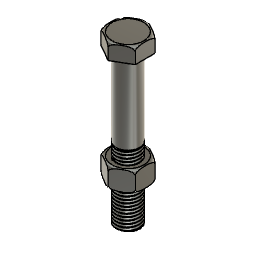
Part 5_ Modelling Features v2 (Autodesk Fusion 360 design; units mm, degrees)
Autodesk Fusion 360 part; units mm, degrees
sketch "Sketch1" plane through (0, 0, 0) normal (0, 0, 1) x (1, 0, 0)
  circle A0 centre (0, 0) radius 6
  line L0 (0, 10) -> (-8.6603, 5)
  line L1 (-8.6603, 5) -> (-8.6603, -5)
  line L2 (-8.6603, -5) -> (0, -10)
  line L3 (0, -10) -> (8.6603, -5)
  line L4 (8.6603, -5) -> (8.6603, 5)
  line L5 (8.6603, 5) -> (0, 10)
  dimension "d1" = 12
  dimension "d2" = 10
  constraint coincident A0.centre origin
  constraint vertical L4
  measures "d1" diameter of A0
  measures "d2" distance of L0.start A0.centre
extrude "Extrude1" add sketch "Sketch1" along normal blind 76 contours A0 makes body 1
extrude "Extrude2" add sketch "Sketch1" along normal blind 7.6 from surface at 76 contours A0 | L0 L1 L2 L3 L4 L5 bodies 1
sketch "Sketch4" plane through (0, 0, 83.6) normal (0, 0, 1) x (-1, 0, 0)
  line L0 (-8.6603, 5) -> (-8.6603, -5)
  line L1 (-8.6603, -5) -> (0, -10)
  line L2 (0, -10) -> (8.6603, -5)
  line L3 (8.6603, -5) -> (8.6603, 5)
  line L4 (8.6603, 5) -> (0, 10)
  line L5 (0, 10) -> (-8.6603, 5)
  circle A0 centre (0, 0) radius 10
  line L6 (-8.6603, -5) -> (0, -10)
  line L7 (0, -10) -> (8.6603, -5)
  line L8 (8.6603, -5) -> (8.6603, 5)
  line L9 (8.6603, 5) -> (0, 10)
  line L10 (0, 10) -> (-8.6603, 5)
  line L11 (-8.6603, 5) -> (-8.6603, -5)
  constraint coincident A0.centre origin
  constraint coincident L0.end A0
  constraint coincident L0.end L1.start
extrude "Extrude3" add sketch "Sketch4" against normal blind 7.6 bodies 1
fillet "Fillet1" radius 2 1 edges at (9.3233, 3.6162, 83.6) on bodies 1
extrude "Extrude4" cut sketch "Sketch4" against normal blind 7.6 contours L0 L1 L2 L3 L4 L5 L6 L7 L8 L9 L10 L11 keep common part bodies 1
extrude "Extrude5" add sketch "Sketch1" along normal blind 76 contours A0 bodies 1
thread "Thread1" "ISO Metric profile 12.0 M12x1.5 6g" major diameter 11.85 minor diameter 10.137 pitch 1.5 angle 60 modelled right hand crest width 0.2154 on face at (5.9702, -0.5974, 50.6667) from (0, 0, 0) to (0, 0, 36) crest through (5.925, 0, -0.375) on bodies 1
extrude "Extrude6" add sketch "Sketch4" against normal blind 10 from surface at -55 separate body makes body 2
fillet "Fillet2" radius 2 2 edges at (9.3233, 3.6162, 28.6) (9.3233, -3.6162, 18.6) on bodies 2
extrude "Extrude7" cut sketch "Sketch4" against normal blind 80 contours L0 L1 L2 L3 L4 L5 L6 L7 L8 L9 L10 L11 keep common part bodies 2
extrude "Extrude8" cut sketch "Sketch1" along normal blind 60 contours A0 bodies 2
thread "Thread2" "ISO Metric profile 12.0 M12x1.5 6H" major diameter 12.203 minor diameter 10.526 pitch 1.5 angle 60 modelled right hand crest width 0.4065 on face at (5.9925, 0.2991, 21.9333) crest through (5.263, 0, 18.975) on bodies 2
move_body "Move1" bodies 2 to x (1, 0, 0) y (0, 1, 0) z (0, 0, 1) at (0, 0.0311, 0.871)
